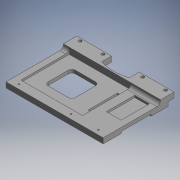
# Autodesk Inventor part: Base Extension 1
Saved by Autodesk Inventor 2020.5 (Build 245400000, 400)
## iProperties
Created: 2023-04-02
Part Number: Base Extension 1
Material: Generic
Document SubType Name: Modeling
Designer: Wes
Density: 1 g/cm^3
Appearance: Default
Author: Wes
Autodesk Inventor part; units mm, degrees
ref_plane "YZ Plane" through (0, 0, 0) normal (1, 0, 0) x (0, 1, 0)
ref_plane "XZ Plane" through (0, 0, 0) normal (0, 1, 0) x (-1, 0, 0)
ref_plane "XY Plane" through (0, 0, 0) normal (0, 0, 1) x (1, 0, 0)
sketch "Sketch1" plane through (0, 0, 0) normal (0, 0, 1) x (1, 0, 0)
  line L0 (0, 0) -> (0, 22.958) construction
  line L1 (0, 0) -> (0, -22.958) construction
  line L2 (0, -22.958) -> (16.63, -22.958) construction
  line L3 (16.63, -22.958) -> (16.63, -81.958) construction
  line L4 (16.63, -81.958) -> (0, -81.958) construction
  line L5 (0, -81.958) -> (0, -22.958) construction
  line L6 (0, 22.958) -> (16.63, 22.958) construction
  line L7 (16.63, 22.958) -> (16.63, 81.958) construction
  line L8 (16.63, 81.958) -> (0, 81.958) construction
  line L9 (0, 81.958) -> (0, 22.958) construction
  line L10 (0, -52.458) -> (0.5, -52.458) construction
  line L11 (8.315, -22.958) -> (8.315, -23.458) construction
  line L12 (0, 0) -> (-53.686, 0) construction
  circle A0 centre (-53.686, 0) radius 74 construction
  line L13 (20.314, 0) -> (20.814, 0) construction
  line L14 (16.63, -22.958) -> (17.13, -22.958) construction
  line L15 (16.63, 22.958) -> (17.13, 22.958) construction
  line L16 (0.5, -23.458) -> (17.13, -23.458)
  line L17 (17.13, -23.458) -> (17.13, -81.958)
  line L18 (17.13, -81.958) -> (0.5, -81.958)
  line L19 (0.5, -81.958) -> (0.5, -23.458)
  line L20 (8.315, 22.958) -> (8.315, 23.458) construction
  line L21 (0.5, 81.958) -> (17.13, 81.958)
  line L22 (17.13, 81.958) -> (17.13, 23.458)
  line L23 (17.13, 23.458) -> (0.5, 23.458)
  line L24 (0.5, 23.458) -> (0.5, 81.958)
  arc A1 (17.13, -23.458) -> (17.13, 23.458) centre (-55.7128, 0) ccw
  line L25 (17.13, -81.958) -> (23.13, -81.958)
  line L26 (23.13, -81.958) -> (23.13, 81.958)
  line L27 (23.13, 81.958) -> (17.13, 81.958)
  dimension "d8" = 148
  dimension "d0" = 22.958
  dimension "d1" = 22.958
  dimension "d2" = 16.63
  dimension "d3" = 59
  dimension "d5" = 0.5
  dimension "d6" = 0.5
  dimension "d7" = 53.686
  dimension "d9" = 0.5
  dimension "d10" = 0.5
  dimension "d11" = 0.5
  dimension "d13" = 0.5
  dimension "d14" = 6
  constraints: 56 end point, 8 horizontal, 8 parallel, 7 perpendicular, 4 vertical, 3 midpoint, 3 point on circle, 2 point on line, 1 centre point, 1 coincident, 1 horizontal alignment, 2 other
  measures "d0" distance of L0.start L0.end
  measures "d1" distance of L0.start L1.end
  measures "d2" distance of L3.end L4.end
  measures "d3" distance of L2.end L3.end
  measures "d5" distance of L10.start L10.end
  measures "d6" distance of L11.start L11.end
  measures "d7" distance of L0.start L12.end
  measures "d9" distance of L13.start L13.end
  measures "d10" distance of L2.end L14.end
  measures "d11" distance of L6.end L15.end
  measures "d13" distance of L20.start L20.end
  measures "d14" distance of L17.end L25.end
extrude "Extrusion1" add sketch "Sketch1" along normal blind 9
sketch "Sketch2" plane through (0, 0, 0) normal (0, 0, -1) x (-1, 0, 0)
  line L0 (-16.63, 22.958) -> (-16.63, 81.958) construction
  circle A0 centre (53.686, 0) radius 74 construction
  line L1 (-16.63, -22.958) -> (-16.63, -81.958) construction
  line L2 (-0.5, 23.458) -> (-17.13, 23.458) projected
  line L3 (-16.63, 23.458) -> (-16.63, 81.958)
  line L4 (-23.13, 81.958) -> (-0.5, 81.958) projected
  line L5 (-17.13, -23.458) -> (-0.5, -23.458) projected
  line L6 (-16.63, -23.458) -> (-16.63, -81.958)
  line L7 (-0.5, -81.958) -> (-23.13, -81.958) projected
  arc A1 (-17.13, 23.458) -> (-17.13, -23.458) centre (55.7128, 0) ccw projected
  arc A2 (-17.13, 23.458) -> (-17.13, -23.458) centre (55.7128, 0) ccw
  line L8 (-23.13, 81.958) -> (-110.13, 81.958)
  line L9 (-110.13, 81.958) -> (-110.13, -81.958)
  line L10 (-110.13, -81.958) -> (-23.13, -81.958)
  line L11 (-23.13, -81.958) -> (-23.13, 81.958)
  line L12 (0, 0) -> (-10.5, 0) construction
  line L13 (-0.5, -81.958) -> (-23.13, -81.958) projected
  arc A3 (-10.5, 38.3695) -> (-10.5, -38.3695) centre (55.7128, 0) ccw
  line L14 (-10.5, 38.3695) -> (-10.5, 81.958)
  line L15 (-10.5, -38.3695) -> (-10.5, -81.958)
  point P0 (-10, 81.958)
  dimension "d17" = 87
  dimension "d66" = 10.5
  constraints: 18 end point, 7 point on line, 5 perpendicular, 4 point on circle, 2 centre point, 2 horizontal, 2 parallel
  measures "d17" distance of L10.end L9.end
  measures "d66" distance of L12.start L12.end
extrude "Extrusion2" add sketch "Sketch2" along normal blind 7 and the other way blind 2 contours A1 A3 L6 L7 L11 L4 L3 | L3 L4 L14 A3 | A3 L15 L7 L6 | L11 L10 L9 L8
sketch "Sketch3" plane through (0, 0, 9) normal (0, 0, 1) x (1, 0, 0)
  line L0 (0.5, -81.958) -> (23.13, -81.958) construction
  line L1 (0, -23.458) -> (10, -23.458) construction
  line L2 (10, -23.458) -> (10, -81.958) construction
  line L3 (10, -81.958) -> (0, -81.958) construction
  line L4 (0, -81.958) -> (0, -23.458) construction
  line L5 (0, 23.458) -> (10, 23.458) construction
  line L6 (0, 81.958) -> (0, 23.458) construction
  line L7 (5, -81.958) -> (5, -71.958) construction
  line L8 (17.13, -23.458) -> (0.5, -23.458) construction
  line L9 (5, -23.458) -> (5, -33.458) construction
  line L10 (5, -23.458) -> (15, -23.458) construction
  circle A0 centre (5, -71.958) radius 1.75
  circle A1 centre (5, -33.458) radius 1.75
  line L11 (-21.548, 0) -> (41.2165, 0) construction
  circle A2 centre (5, 71.958) radius 1.75
  circle A3 centre (5, 33.458) radius 1.75
  point P0 (0, 0)
  dimension "d20" = 10
  dimension "d21" = 10
  dimension "d22" = 10
  dimension "d24" = 3.5
  dimension "d25" = 3.5
  constraints: 20 end point, 4 centre point, 4 horizontal, 3 perpendicular, 2 coincident, 2 parallel, 2 point on line, 2 symmetric about line, 1 midpoint, 1 vertical, 2 other
  measures "d20" distance of L2.end L3.end
  measures "d21" distance of L7.start L7.end
  measures "d22" distance of L9.start L9.end
  measures "d24" diameter of A0
  measures "d25" diameter of A1
extrude "Extrusion3" cut sketch "Sketch3" against normal up to surface (9 mm away)
sketch "Sketch4" plane through (0, 0, 9) normal (0, 0, 1) x (1, 0, 0)
  circle A0 centre (5, -71.958) radius 1.75 projected
  circle A1 centre (5, -71.958) radius 2.65
  circle A2 centre (5, -33.458) radius 1.75 projected
  circle A3 centre (5, -33.458) radius 2.65
  circle A4 centre (5, 33.458) radius 1.75 projected
  circle A5 centre (5, 33.458) radius 2.65
  circle A6 centre (5, 71.958) radius 1.75 projected
  circle A7 centre (5, 71.958) radius 2.65
  point P0 (0, 0)
  dimension "d28" = 5.3
  dimension "d29" = 5.3
  constraints: 4 centre point, 4 coincident
  measures "d28" diameter of A1
  measures "d29" diameter of A3
extrude "Extrusion4" cut sketch "Sketch4" against normal blind 6 contours A0 | A1 | A2 | A3 | A4 | A5 | A6 | A7
sketch "Sketch5" plane through (0, 0, 2) normal (0, 0, 1) x (1, 0, 0)
  line L0 (23.13, -71.958) -> (105.13, -71.958)
  line L1 (105.13, -71.958) -> (105.13, 32.042)
  line L2 (105.13, 32.042) -> (23.13, 32.042)
  line L3 (23.13, 32.042) -> (23.13, -71.958)
  line L4 (31.2383, 46.3792) -> (79.2383, 46.3792)
  line L5 (79.2383, 46.3792) -> (79.2383, 71.3792)
  line L6 (79.2383, 71.3792) -> (31.2383, 71.3792)
  line L7 (31.2383, 71.3792) -> (31.2383, 46.3792)
  line L8 (23.13, -81.958) -> (23.13, 81.958) construction
  line L9 (23.13, -81.958) -> (23.13, 81.958) construction
  line L10 (23.13, -81.958) -> (23.13, -71.958) construction
  point P0 (0, 0)
  dimension "d34" = 82
  dimension "d35" = 104
  dimension "d36" = 48
  dimension "d37" = 25
  dimension "d38" = 10
  constraints: 20 end point, 4 parallel, 2 horizontal, 2 perpendicular, 1 collinear, 1 point on line
  measures "d34" distance of L2.end L1.end
  measures "d35" distance of L1.end L0.end
  measures "d36" distance of L6.end L5.end
  measures "d37" distance of L5.end L4.end
  measures "d38" distance of L8.start L10.end
extrude "Extrusion5" cut sketch "Sketch5" against normal blind 3.5
sketch "Sketch6" plane through (0, 0, 2) normal (0, 0, 1) x (1, 0, 0)
  line L0 (23.13, 32.042) -> (105.13, 32.042) projected
  line L1 (64.13, 32.042) -> (39.13, 32.042)
  line L2 (64.13, 32.042) -> (89.13, 32.042)
  line L3 (89.13, 32.042) -> (89.13, 25.042)
  line L4 (89.13, 25.042) -> (39.13, 25.042)
  line L5 (39.13, 25.042) -> (39.13, 32.042)
  point P0 (0, 0)
  dimension "d41" = 25
  dimension "d42" = 25
  dimension "d43" = 7
  constraints: 10 end point, 2 point on line, 1 midpoint, 1 parallel, 1 perpendicular, 1 vertical
  measures "d41" distance of L1.start L1.end
  measures "d42" distance of L1.start L2.end
  measures "d43" distance of L2.end L3.end
extrude "Extrusion6" cut sketch "Sketch6" against normal up to surface (9 mm away)
sketch "Sketch7" plane through (23.13, 32.042, 2) normal (0, -1, 0) x (1, 0, 0)
  line L0 (66, -9) -> (16, -9) projected
  line L1 (66, -3.5) -> (66, -9) projected
  line L2 (16, -9) -> (66, -9)
  line L3 (66, -9) -> (66, -6)
  line L4 (66, -6) -> (16, -6)
  line L5 (16, -6) -> (16, -9)
  point P0 (-23.13, -2)
  dimension "d46" = 3
  constraints: 8 end point, 2 parallel, 1 horizontal, 1 perpendicular, 1 point on line
  measures "d46" distance of L3.end L2.end
extrude "Extrusion7" cut sketch "Sketch7" against normal up to surface (49.916 mm away)
sketch "Sketch8" plane through (0, 0, -1.5) normal (0, 0, 1) x (1, 0, 0)
  line L0 (41.13, -49.8888) -> (87.13, -49.8888)
  line L1 (87.13, -49.8888) -> (87.13, -3.8888)
  line L2 (87.13, -3.8888) -> (41.13, -3.8888)
  line L3 (41.13, -3.8888) -> (41.13, -49.8888)
  line L4 (41.13, -49.8888) -> (87.13, -3.8888) construction
  line L5 (87.13, -49.8888) -> (41.13, -3.8888) construction
  point P0 (0, 0)
  point P1 (64.13, -26.8888)
  dimension "d49" = 46
  dimension "d50" = 46
  constraints: 12 end point, 2 midpoint, 2 parallel, 1 horizontal, 1 perpendicular
  measures "d49" distance of L2.end L1.end
  measures "d50" distance of L1.end L0.end
extrude "Extrusion8" cut sketch "Sketch8" against normal up to surface (5.5 mm away)
sketch "Sketch9" plane through (0, 0, 2) normal (0, 0, 1) x (1, 0, 0)
  line L0 (110.13, 81.958) -> (110.13, -81.958) projected
  line L1 (110.13, -81.958) -> (120.13, -81.958)
  line L2 (120.13, -81.958) -> (120.13, 81.958)
  line L3 (120.13, 81.958) -> (110.13, 81.958)
  line L4 (110.13, 81.958) -> (110.13, -81.958)
  point P0 (0, 0)
  dimension "d53" = 10
  constraints: 8 end point, 2 parallel, 1 horizontal, 1 perpendicular
  measures "d53" distance of L3.end L2.end
extrude "Extrusion9" add sketch "Sketch9" against normal blind 9
sketch "Sketch10" plane through (0, 0, 2) normal (0, 0, 1) x (1, 0, 0)
  line L0 (105.13, 32.042) -> (105.13, -71.958) construction
  line L1 (105.13, -71.958) -> (120.13, -71.958) construction
  line L2 (120.13, -81.958) -> (120.13, 81.958) construction
  circle A0 centre (112.63, -67.7077) radius 1.275
  circle A1 centre (112.63, 66.21) radius 1.275
  circle A2 centre (112.63, 20.0315) radius 1.275
  line L3 (23.13, -81.958) -> (120.13, -81.958) construction
  line L4 (112.63, 66.21) -> (112.63, 81.958) construction
  line L5 (89.13, 81.958) -> (120.13, 81.958) construction
  line L6 (112.63, 66.21) -> (112.63, 20.0315) construction
  line L7 (112.63, -67.7077) -> (112.63, -81.958) construction
  point P0 (0, 0)
  dimension "d56" = 2.55
  dimension "d57" = 2.55
  dimension "d58" = 2.55
  dimension "d60" = 15.748
  dimension "d61" = 46.1785
  dimension "d62" = 14.2503
  constraints: 8 end point, 3 centre point, 3 point on line, 2 vertical, 1 horizontal, 1 perpendicular
  measures "d56" diameter of A0
  measures "d57" diameter of A1
  measures "d58" diameter of A2
  measures "d60" distance of L4.start L4.end
  measures "d61" distance of L4.start L6.end
  measures "d62" distance of L7.start L7.end
extrude "Extrusion10" cut sketch "Sketch10" against normal blind 4.5
fillet "Fillet1" radius 6 6 edges at (41.13, -49.8888, -4.25) (41.13, -3.8888, -4.25) (87.13, -3.8888, -4.25) (87.13, -49.8888, -4.25) (23.13, -76.958, 2) (23.13, 57, 2)
body "Solid1"
